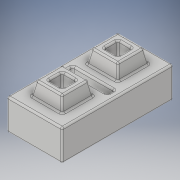
# Autodesk Inventor part: cap stone 2.0
Saved by Autodesk Inventor 2019 (Build 230136000, 136)
## iProperties
Created: 2019-12-02
Part Number: cap stone 2.0
Material: Generic
Document SubType Name: Modeling
Designer: User
Density: 1 g/cm^3
Appearance: Default
Author: User
Autodesk Inventor part; units mm, degrees
ref_plane "YZ Plane" through (0, 0, 0) normal (1, 0, 0) x (0, 1, 0)
ref_plane "XZ Plane" through (0, 0, 0) normal (0, 1, 0) x (-1, 0, 0)
ref_plane "XY Plane" through (0, 0, 0) normal (0, 0, 1) x (1, 0, 0)
sketch "Sketch1" plane through (0, 0, 0) normal (0, 1, 0) x (-1, 0, 0)
  line L0 (50.8, -101.6) -> (-50.8, -101.6)
  line L1 (-50.8, -101.6) -> (-50.8, 101.6)
  line L2 (-50.8, 101.6) -> (50.8, 101.6)
  line L3 (50.8, 101.6) -> (50.8, -101.6)
  line L4 (50.8, -101.6) -> (-50.8, 101.6) construction
  line L5 (-50.8, -101.6) -> (50.8, 101.6) construction
  line L6 (-28.575, 79.375) -> (28.575, 79.375)
  line L7 (28.575, 79.375) -> (28.575, 22.225)
  line L8 (28.575, 22.225) -> (-28.575, 22.225)
  line L9 (-28.575, 22.225) -> (-28.575, 79.375)
  line L10 (-28.575, 79.375) -> (28.575, 22.225) construction
  line L11 (28.575, 79.375) -> (-28.575, 22.225) construction
  line L12 (-28.575, -79.375) -> (28.575, -79.375)
  line L13 (28.575, -79.375) -> (28.575, -22.225)
  line L14 (28.575, -22.225) -> (-28.575, -22.225)
  line L15 (-28.575, -22.225) -> (-28.575, -79.375)
  line L16 (-28.575, -79.375) -> (28.575, -22.225) construction
  line L17 (28.575, -79.375) -> (-28.575, -22.225) construction
  point P0 (0, 0)
  point P1 (0, 50.8)
  point P2 (0, -50.8)
  dimension "d0" = 101.6
  dimension "d1" = 203.2
  dimension "d2" = 57.15
  dimension "d3" = 57.15
  dimension "d4" = 57.15
  dimension "d5" = 57.15
  dimension "d6" = 0
  dimension "d7" = 50.8
  dimension "d8" = 50.8
  constraints: 36 end point, 6 midpoint, 6 parallel, 3 horizontal, 3 perpendicular, 1 point on line
  measures "d0" distance of L1.end L2.end
  measures "d1" distance of L0.end L1.end
  measures "d2" distance of L12.start L12.end
  measures "d3" distance between parallel lines of L14 L12
  measures "d4" distance of L6.start L6.end
  measures "d5" distance between parallel lines of L8 L6
  measures "d6" horizontal distance of point (0, 0) point (0, 50.8)
  measures "d7" distance of point (0, 0) point (0, 50.8)
  measures "d8" distance of point (0, 0) point (0, -50.8)
extrude "Extrusion1" add sketch "Sketch1" along normal blind 38.1
sketch "Sketch2" plane through (0, 38.1, 0) normal (0, 1, 0) x (1, 0, 0)
  line L0 (50.8, 101.6) -> (-50.8, 101.6) projected
  line L1 (50.8, -101.6) -> (-50.8, -101.6)
  line L2 (-50.8, -101.6) -> (-50.8, 101.6)
  line L3 (-50.8, 101.6) -> (50.8, 101.6)
  line L4 (50.8, 101.6) -> (50.8, -101.6)
  line L5 (50.8, -101.6) -> (-50.8, 101.6) construction
  line L6 (-50.8, -101.6) -> (50.8, 101.6) construction
  point P0 (0, 0)
  constraints: 12 end point, 2 midpoint, 2 parallel, 1 horizontal, 1 perpendicular
extrude "Extrusion2" add sketch "Sketch2" along normal blind 19.05
sketch "Sketch3" plane through (0, 57.15, 0) normal (0, 1, 0) x (1, 0, 0)
  line L0 (-28.575, -79.375) -> (28.575, -79.375) projected
  line L1 (-28.575, -22.225) -> (-28.575, -79.375) projected
  line L2 (-28.575, -79.375) -> (-28.575, -22.225)
  line L3 (28.575, -79.375) -> (28.575, -22.225) projected
  line L4 (-28.575, -22.225) -> (28.575, -22.225)
  line L5 (28.575, -22.225) -> (28.575, -79.375)
  line L6 (28.575, -79.375) -> (-28.575, -79.375)
  line L7 (28.575, 22.225) -> (-28.575, 22.225) projected
  line L8 (28.575, 22.225) -> (-28.575, 22.225)
  line L9 (-28.575, 79.375) -> (-28.575, 22.225) projected
  line L10 (-28.575, 22.225) -> (-28.575, 79.375)
  line L11 (28.575, 79.375) -> (-28.575, 79.375) projected
  line L12 (-28.575, 79.375) -> (28.575, 79.375)
  line L13 (28.575, 79.375) -> (28.575, 22.225) projected
  line L14 (28.575, 79.375) -> (28.575, 22.225)
  point P0 (0, 0)
  constraints: 16 end point, 4 perpendicular, 3 collinear, 1 vertical
extrude "Extrusion4" add sketch "Sketch3" along normal blind 25.4 draft -10.619
fillet "Fillet1" radius 3.175 60 edges at (28.575, 57.15, 50.8) (0, 57.15, 79.375) (23.8128, 82.55, 50.8) (0, 82.55, 74.6128) (26.1939, 69.85, 76.9939) (26.1939, 69.85, 24.6061) (-26.1939, 69.85, 24.6061) (0, 57.15, 22.225) (-28.575, 57.15, 50.8) (-23.8128, 82.55, 50.8) (0, 82.55, 26.9872) (-23.8128, 82.55, -50.8) (0, 82.55, -74.6128) (23.8128, 82.55, -50.8) (0, 82.55, -26.9872) (0, 57.15, -22.225) (28.575, 57.15, -50.8) (26.1939, 69.85, -24.6061) (26.1939, 69.85, -76.9939) (50.8, 0, 0) (-26.1939, 69.85, -76.9939) (0, 57.15, -79.375) (-28.575, 57.15, -50.8) (-50.8, 57.15, 0) (0, 57.15, -101.6) (-50.8, 28.575, -101.6) (-50.8, 0, 0) (0, 0, -101.6) (-50.8, 28.575, 101.6) (0, 57.15, 101.6) (0, 0, 101.6) (50.8, 57.15, 0) (50.8, 28.575, -101.6) (0, 0, -22.225) (0, 38.1, -22.225) (28.575, 19.05, -22.225) (28.575, 38.1, -50.8) (28.575, 0, -50.8) (0, 0, -79.375) (-28.575, 0, -50.8) (28.575, 38.1, 50.8) (0, 38.1, 79.375) (28.575, 19.05, 79.375) (0, 0, 22.225) (28.575, 0, 50.8) (0, 0, 79.375) (-28.575, 0, 50.8) (-28.575, 38.1, -50.8) (-28.575, 19.05, -79.375) (0, 38.1, -79.375) (-28.575, 19.05, 22.225) (-28.575, 38.1, 50.8) (0, 38.1, 22.225) (-28.575, 19.05, -22.225) (-28.575, 19.05, 79.375) (28.575, 19.05, 22.225) (28.575, 19.05, -79.375) (50.8, 28.575, 101.6) (-26.1939, 69.85, 76.9939) (-26.1939, 69.85, -24.6061)
sketch "Sketch7" plane through (0, 82.55, 0) normal (0, 1, 0) x (1, 0, 0)
  line L0 (-12.7, 38.1) -> (12.7, 38.1)
  line L1 (12.7, 38.1) -> (12.7, 63.5)
  line L2 (12.7, 63.5) -> (-12.7, 63.5)
  line L3 (-12.7, 63.5) -> (-12.7, 38.1)
  line L4 (-12.7, 38.1) -> (12.7, 63.5) construction
  line L5 (12.7, 38.1) -> (-12.7, 63.5) construction
  line L6 (12.7, -38.1) -> (-12.7, -38.1)
  line L7 (-12.7, -38.1) -> (-12.7, -63.5)
  line L8 (-12.7, -63.5) -> (12.7, -63.5)
  line L9 (12.7, -63.5) -> (12.7, -38.1)
  line L10 (12.7, -38.1) -> (-12.7, -63.5) construction
  line L11 (-12.7, -38.1) -> (12.7, -63.5) construction
  point P0 (0, 0)
  point P1 (0, 50.8)
  point P2 (0, -50.8)
  dimension "d42" = 25.4
  dimension "d43" = 25.4
  dimension "d44" = 0
  dimension "d45" = 50.8
  dimension "d46" = 25.4
  dimension "d47" = 25.4
  dimension "d48" = 0
  dimension "d49" = 50.8
  constraints: 24 end point, 4 midpoint, 4 parallel, 2 horizontal, 2 perpendicular
  measures "d42" distance of L2.end L1.end
  measures "d43" distance of L1.end L0.end
  measures "d44" horizontal distance of point (0, 0) point (0, 50.8)
  measures "d45" distance of point (0, 0) point (0, 50.8)
  measures "d46" distance of L8.end L7.end
  measures "d47" distance of L7.end L6.end
  measures "d48" horizontal distance of point (0, 0) point (0, -50.8)
  measures "d49" distance of point (0, -50.8) point (0, 0)
extrude "Extrusion5" cut sketch "Sketch7" against normal blind 76.2
sketch "Sketch13" plane through (0, 57.15, 0) normal (0, 1, 0) x (1, 0, 0)
  line L0 (-38.1, 6.35) -> (38.1, 6.35)
  line L1 (38.1, 6.35) -> (38.1, -6.35)
  line L2 (38.1, -6.35) -> (-38.1, -6.35)
  line L3 (-38.1, -6.35) -> (-38.1, 6.35)
  line L4 (-38.1, 6.35) -> (38.1, -6.35) construction
  line L5 (38.1, 6.35) -> (-38.1, -6.35) construction
  point P0 (0, 0)
  dimension "d93" = 76.2
  dimension "d94" = 12.7
  constraints: 12 end point, 2 midpoint, 2 parallel, 1 horizontal, 1 perpendicular
  measures "d93" distance between parallel lines of L3 L1
  measures "d94" distance between parallel lines of L0 L2
extrude "Extrusion11" cut sketch "Sketch13" against normal blind 57.15
fillet "Fillet2" radius 3.175 24 edges at (-12.7, 82.55, 50.8) (0, 82.55, 38.1) (12.7, 82.55, 50.8) (0, 82.55, 63.5) (-12.7, 60.325, 38.1) (12.7, 60.325, 38.1) (12.7, 60.325, 63.5) (-12.7, 60.325, 63.5) (0, 38.1, 63.5) (12.7, 38.1, 50.8) (0, 38.1, 38.1) (-12.7, 38.1, 50.8) (-12.7, 38.1, -50.8) (0, 38.1, -38.1) (0, 38.1, -63.5) (12.7, 38.1, -50.8) (0, 82.55, -63.5) (-12.7, 82.55, -50.8) (-12.7, 60.325, -63.5) (-12.7, 60.325, -38.1) (12.7, 60.325, -38.1) (12.7, 60.325, -63.5) (0, 82.55, -38.1) (12.7, 82.55, -50.8)
fillet "Fillet3" radius 3.175 12 edges at (0, 57.15, 6.35) (0, 57.15, -6.35) (38.1, 57.15, 0) (-38.1, 57.15, 0) (-38.1, 28.575, 6.35) (38.1, 28.575, 6.35) (38.1, 28.575, -6.35) (-38.1, 28.575, -6.35) (38.1, 0, 0) (0, 0, 6.35) (0, 0, -6.35) (-38.1, 0, 0)
equation "\"d8\" = d7"
equation "\"d49\" = d45"
body "Solid1"
